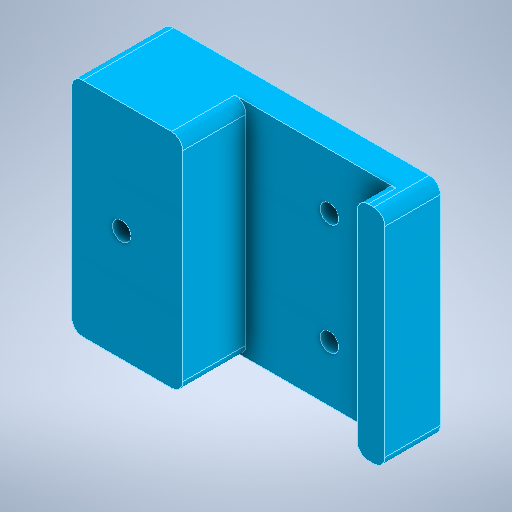
# Autodesk Inventor part: soroban_hold
Saved by Autodesk Inventor 2025.1 (Build 291241000, 241)
## iProperties
Created: 2024-10-17
Part Number: soroban_hold
Material: 一般
Document SubType Name: Modeling
Designer: yuki0520
Density: 1 g/cm^3
Appearance: スカイ ブルー 標準
Author: yuki0520
Autodesk Inventor part; units mm, degrees
ref_plane "YZ Plane" through (0, 0, 0) normal (1, 0, 0) x (0, 1, 0)
ref_plane "XZ Plane" through (0, 0, 0) normal (0, 1, 0) x (-1, 0, 0)
ref_plane "XY Plane" through (0, 0, 0) normal (0, 0, 1) x (1, 0, 0)
sketch "スケッチ1" plane through (0, 0, 0) normal (0, 0, 1) x (1, 0, 0)
  line L0 (22.5, -20) -> (-22.5, -20)
  line L1 (-22.5, -20) -> (-22.5, 20)
  line L2 (-22.5, 20) -> (22.5, 20)
  line L3 (22.5, 20) -> (22.5, -20)
  line L4 (22.5, -20) -> (-22.5, 20) construction
  line L5 (-22.5, -20) -> (22.5, 20) construction
  circle A0 centre (12.5, 10) radius 1.65
  circle A1 centre (12.5, -10) radius 1.65
  circle A2 centre (-13.5, 0) radius 1.65
  point P0 (0, 0)
  dimension "d0" = 45
  dimension "d1" = 40
  dimension "d2" = 3.3
  dimension "d3" = 3.3
  dimension "d4" = 10
  dimension "d5" = 10
  dimension "d6" = 10
  dimension "d7" = 10
  dimension "d8" = 3.3
  dimension "d9" = 36
  dimension "d10" = 20
  constraints: 12 end point, 3 centre point, 2 midpoint, 2 parallel, 1 horizontal, 1 perpendicular
  measures "d0" distance of L1.end L2.end
  measures "d1" distance of L0.end L1.end
  measures "d2" diameter of A0
  measures "d3" diameter of A1
  measures "d4" distance from line of L3 A0.centre
  measures "d5" distance from line of L3 A1.centre
  measures "d6" distance from line of L2 A0.centre
  measures "d7" distance from line of L0 A1.centre
  measures "d8" diameter of A2
  measures "d9" distance from line of L3 A2.centre
  measures "d10" distance from line of L2 A2.centre
extrude "押し出し1" add sketch "スケッチ1" along normal blind 5
sketch "スケッチ2" plane through (0, 0, 5) normal (0, 0, 1) x (1, 0, 0)
  line L0 (22.5, 20) -> (-22.5, 20) projected
  line L1 (-22.5, 20) -> (-22.5, -20) projected
  line L2 (-22.5, -20) -> (22.5, -20) projected
  line L3 (22.5, -20) -> (22.5, 20) projected
  circle A0 centre (-13.5, 0) radius 1.65 projected
  circle A1 centre (12.5, -10) radius 1.65 projected
  circle A2 centre (12.5, 10) radius 1.65 projected
  line L4 (-22.5, 20) -> (0, 20)
  line L5 (0, 20) -> (0, -20)
  line L6 (0, -20) -> (-22.5, -20)
  line L7 (-22.5, -20) -> (-22.5, 20)
  line L8 (22.5, 20) -> (-22.5, 20) projected
  line L9 (-2.5, 20) -> (-2.5, -20)
  point P0 (0, 0)
  point P1 (-2.5, -20)
  dimension "d15" = 20
  constraints: 10 end point, 2 parallel, 2 perpendicular, 2 point on line, 1 horizontal, 1 midpoint
  measures "d15" distance between parallel lines of L1 L9
extrude "押し出し2" add sketch "スケッチ2" along normal blind 11.4 contours L9 L2 L1 L0
fillet "フィレット1" radius 2 4 edges at (-22.5, 20, 8.2) (-22.5, -20, 8.2) (-2.5, -20, 10.7) (-2.5, 20, 10.7)
sketch "スケッチ3" plane through (22.5, -20, 0) normal (1, 0, 0) x (0, 0, -1)
  line L0 (0, 0) -> (0, 40) projected
  line L1 (0, 40) -> (-5, 40) projected
  line L2 (-5, 0) -> (-5, 40) projected
  line L3 (0, 0) -> (-5, 0) projected
  line L4 (-5, 40) -> (-16.4, 40) projected
  line L5 (0, 0) -> (-10, 0)
  line L6 (-10, 0) -> (-10, 40)
  line L7 (-10, 40) -> (0, 40)
  line L8 (0, 40) -> (0, 0)
  point P0 (0, 20)
  dimension "d17" = 10
  constraints: 8 end point, 2 parallel, 1 horizontal, 1 perpendicular, 1 point on line
  measures "d17" distance of L6.end L7.end
extrude "押し出し3" add sketch "スケッチ3" along normal blind 5
fillet "フィレット2" radius 2 4 edges at (27.5, 20, 5) (27.5, -20, 5) (22.5, 20, 7.5) (22.5, -20, 7.5)
